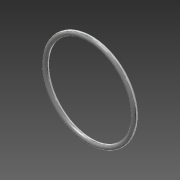
# Autodesk Inventor part: Ciąg
Saved by Autodesk Inventor 2015 (Build 190159000, 159)
## iProperties
Created: 2016-01-12
Part Number: Ciąg
Material: Aluminium 6061-AHC
Document SubType Name: Modeling
Designer: graaapsik
Density: 2.71 g/cm^3
Appearance: Aluminium - ciemne
Mass: 842.519 g
Surface Area: 3108.93 cm^2
Volume: 310.893 cm^3
Author: graaapsik
Autodesk Inventor part; units mm, degrees
ref_plane "YZ Plane" through (0, 0, 0) normal (1, 0, 0) x (0, 1, 0)
ref_plane "XZ Plane" through (0, 0, 0) normal (0, 1, 0) x (-1, 0, 0)
ref_plane "XY Plane" through (0, 0, 0) normal (0, 0, 1) x (1, 0, 0)
sketch "Szkic1" plane through (0, 0, 0) normal (1, 0, 0) x (0, 1, 0)
  circle A0 centre (0, 281.25) radius 15
  circle A1 centre (0, 281.25) radius 13
  line L0 (-84.8352, 0) -> (115.9844, 0)
  point P0 (0, 0)
  dimension "d0" = 30
  dimension "d1" = 2
  dimension "d2" = 281.25
  constraints: 2 centre point, 2 end point, 1 horizontal, 1 vertical alignment
  measures "d0" diameter of A0
  measures "d1" radial gap between concentric circles of A0 A1
  measures "d2" distance of point (0, 0) A0.centre
revolve "Obrót1" add sketch "Szkic1" angle 360 about axis through (0, -84.8352, 0) along (0, 1, 0)
